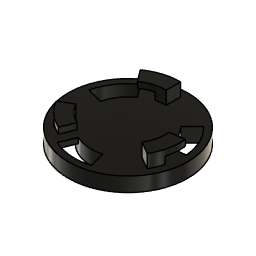
Pièce reliant LiDAR et robot v15 (Autodesk Fusion 360 design; units mm, degrees)
Autodesk Fusion 360 part; units mm, degrees
sketch "Esquisse2" plane through (0, 0, 0) normal (0, 0, 1) x (1, 0, 0) in component "Cercle 50mm"
  circle A0 centre (0, 0) radius 25
  line L0 (0, 22) -> (0, 16)
  line L1 (-21.2504, 5.694) -> (-19.9976, 10.3696) construction
  line L2 (-21.2504, 5.694) -> (-15.4548, 4.1411)
  arc A1 (0, 16) -> (-9.4683, 12.8977) centre (0, 0) ccw
  arc A2 (0, 22) -> (-13.1215, 17.6586) centre (0, 0) ccw
  line L3 (-13.1215, 17.6586) -> (-9.4683, 12.8977)
  line L4 (-5.694, 21.2504) -> (-1.6075, 22.3454) construction
  line L5 (-5.694, 21.2504) -> (-4.1411, 15.4548)
  arc A3 (-13.1215, 17.6586) -> (-21.2504, 5.694) centre (0, 0) ccw
  arc A4 (-9.4683, 12.8977) -> (-15.4548, 4.1411) centre (0, 0) ccw
  line L6 (-13.0418, 18.2118) -> (-8.899, 12.8128)
  arc A5 (-8.899, 12.8128) -> (-15.167, 3.6499) centre (0, 0) ccw
  line L7 (-21.7368, 5.4102) -> (-15.167, 3.6499)
  arc A6 (-13.0418, 18.2118) -> (-21.7368, 5.4102) centre (0, 0) ccw
  line L8 (-13.365, 17.976) -> (-9.2248, 12.5803)
  arc A7 (0.4, 22.3964) -> (-13.0857, 18.1804) centre (0, 0) ccw
  line L9 (0.4, 22.3964) -> (0.4, 15.5949)
  arc A8 (0.4, 15.5949) -> (-12.1027, 9.843) centre (0, 0) ccw
  arc A9 (-8.732, -20.1929) -> (5.694, -21.2504) centre (0, 0) ccw
  arc A10 (-6.6467, -14.1132) -> (4.4226, -14.96) centre (0, 0) ccw
  line L10 (5.694, -21.2504) -> (1.0185, -22.5032) construction
  arc A11 (-9.251, -20.4005) -> (6.183, -21.5298) centre (0, 0) ccw
  line L11 (6.183, -21.5298) -> (4.4226, -14.96)
  line L12 (-15.5563, -15.5563) -> (-18.5479, -12.5648) construction
  arc A12 (-13.7056, -7.451) -> (-2.4729, -15.4027) centre (0, 0) ccw
  line L13 (-19.0526, -11) -> (-13.8564, -8)
  line L14 (-19.5959, -10.8518) -> (-13.7056, -7.451)
  line L15 (5.694, -21.2504) -> (4.1411, -15.4548)
  line L16 (-8.8851, -20.5624) -> (-6.2825, -14.279)
  arc A13 (-13.8564, -8) -> (-6.4356, -14.6487) centre (0, 0) ccw
  line L17 (-9.251, -20.4005) -> (-6.6467, -14.1132)
  arc A14 (-19.5959, -10.8518) -> (-9.2018, -20.4227) centre (0, 0) ccw
  arc A15 (-6.4356, -14.6487) -> (4.1411, -15.4548) centre (0, 0) ccw
  line L18 (-8.732, -20.1929) -> (-6.4356, -14.6487)
  line L19 (-15.5563, -15.5563) -> (-11.3137, -11.3137)
  arc A16 (-19.0526, -11) -> (-8.732, -20.1929) centre (0, 0) ccw
  arc A17 (21.8535, 2.5343) -> (15.5563, 15.5564) centre (0, 0) ccw
  arc A18 (15.5457, 1.3004) -> (10.7444, 11.3101) centre (0, 0) ccw
  line L20 (15.5563, 15.5564) -> (18.9791, 12.1336) construction
  arc A19 (22.2928, 2.1886) -> (15.5538, 16.1195) centre (0, 0) ccw
  line L21 (15.5538, 16.1195) -> (10.7444, 11.3101)
  line L22 (21.2504, -5.694) -> (20.1554, -9.7806) construction
  arc A20 (13.3056, -8.1438) -> (14.5756, 5.5597) centre (0, 0) ccw
  line L23 (19.0526, -11) -> (13.8564, -8)
  line L24 (19.1959, -11.5446) -> (13.3056, -8.1438)
  line L25 (15.5563, 15.5564) -> (11.3137, 11.3137)
  line L26 (22.2502, 2.5865) -> (15.5072, 1.6987)
  arc A21 (13.8564, -8) -> (15.9039, 1.751) centre (0, 0) ccw
  line L27 (22.2928, 2.1886) -> (15.5457, 1.3004)
  arc A22 (19.1959, -11.5446) -> (22.2875, 2.2423) centre (0, 0) ccw
  arc A23 (15.9039, 1.751) -> (11.3137, 11.3137) centre (0, 0) ccw
  line L28 (21.8535, 2.5343) -> (15.9039, 1.751)
  line L29 (21.2504, -5.694) -> (15.4548, -4.1411)
  arc A24 (19.0526, -11) -> (21.8535, 2.5343) centre (0, 0) ccw
  dimension "d233" = 50
  dimension "d235" = 6
  dimension "d237" = 75
  dimension "d238" = 3
  dimension "d239" = 15
  dimension "d240" = 37.5
  dimension "d241" = 14.4648
  dimension "d242" = -0.4
  dimension "d243" = 0.4
  dimension "d245" = 360
  dimension "d267" = 0.4
  constraint coincident A0.centre A1.centre
  constraint vertical L0
  constraint coincident L0 A0.centre
  constraint tangent L1 A2
  constraint perpendicular L1 L2
  constraint concentric A0 A1
  constraint concentric A0 A2
  constraint tangent A2 L4
  constraint coincident A2 L4.start
  constraint coincident A1 L5.end
  constraint perpendicular L4 L5
  constraint concentric A2 A3
  constraint concentric A1 A4
  constraint coincident A6 L8.start
  constraint coincident A5 L8.end
  constraint collinear L3 L8
  measures "d233" diameter of A0
  measures "d235" distance of L0.start L0.end
  measures "d237" angle of L0 L2
  measures "d238" distance of A0 A2
  measures "d239" angle of L0 L5
  measures "d240" angle of L2 L3
  measures "d241" distance of L1.start A2.end
  measures "d267" distance of A20 A21
extrude "Extrusion1" add sketch "Esquisse2" along normal blind 2.2 from surface at 2.8 contours A13 L17 L19 A16 | A12 L13 L14 A13 L17 A14 A16 | L13 A13 L19 A16 makes body 1 in component "Cercle 50mm"
extrude "Extrusion2" add sketch "Esquisse2" along normal blind 2.8 from surface at 5 contours L13 A13 L19 A16 bodies 1 in component "Cercle 50mm"
extrude "Extrusion7" add 1 faces at (-16.9768, -10.5396, 7.8) along direction (0, 0, 1) blind 0.7 on bodies 1 bodies 1 in component "Cercle 50mm"
extrude "Extrusion8" cut 1 faces at (-16.9768, -10.5396, 8.5) along direction (0, 0, -1) blind 0.2 on bodies 1 bodies 1 in component "Cercle 50mm"
extrude "Extrusion9" cut 1 faces at (-16.9768, -10.5396, 8.3) along direction (0, 0, -1) blind 0.3 on bodies 1 bodies 1 in component "Cercle 50mm"
extrude "Extrusion10" add sketch "Esquisse2" along normal blind 2.5 from surface at 8 contours A13 L17 L19 A16 | L13 A13 L19 A16 bodies 1 in component "Cercle 50mm"
move_body "Déplacer1" bodies 1 to x (1, 0, 0) y (0, 1, 0) z (0, 0, 1) at (0, 0, 1) in component "Cercle 50mm"
pattern_circular "Réseau C1" count 3 over 360 about axis through (0, 0, 1.75) along (0, 0, 1) of bodies 1 makes body 2 at (20.0762, 0.939, 3.8) makes body 3 at (-10.8513, 16.9169, 3.8) in component "Cercle 50mm"
extrude "Extrusion4" add sketch "Esquisse2" along normal blind 5 bodies 1 2 3 in component "Cercle 50mm"
extrude "Extrusion6" add 1 faces at (5.5148, 3.0091, 5) along direction (0, 0, 1) blind 1 on bodies 1 bodies 1 in component "Cercle 50mm"
component "Cercle 50mm" placed x (1, 0, 0) y (0, 1, 0) z (0, 0, 1) at (0, 0, 0)
